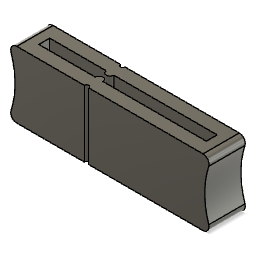
Cassette_Sleeve (Autodesk Fusion 360 design; units mm, degrees)
Autodesk Fusion 360 part; units mm, degrees
sketch "Sketch1" plane through (0, 0, 0) normal (0, 1, 0) x (1, 0, 0)
  line L0 (0, 0) -> (33.75, 0)
  line L1 (33.75, 0) -> (33.75, -6)
  line L2 (33.75, -6) -> (0, -6)
  line L3 (0, -6) -> (0, 0)
  line L4 (3, -3.9) -> (3, -2.1)
  line L5 (30.75, -2.1) -> (30.75, -3.9)
  line L6 (30.75, -3.9) -> (13.625, -3.9)
  line L7 (12.375, -3.9) -> (3, -3.9)
  line L8 (3, -2.1) -> (12.375, -2.1)
  line L9 (13.625, -2.1) -> (30.75, -2.1)
  arc A0 (12.375, -2.1) -> (13.625, -2.1) centre (13, -2.1) ccw
  arc A1 (12.625, 0) -> (13.375, 0) centre (13, 0) ccw
  arc A2 (13.375, -6) -> (12.625, -6) centre (13, -6) ccw
  arc A3 (13.625, -3.9) -> (12.375, -3.9) centre (13, -3.9) ccw
  dimension "d1" = 33.75
  dimension "d2" = 6
  dimension "d8" = 2.1
  dimension "d9" = 3
  dimension "d10" = 2.1
  dimension "d11" = 3
  dimension "d12" = 27
  dimension "d20" = 10
  dimension "d22" = 10
  dimension "d25" = 0.75
  dimension "d26" = 0.75
  dimension "d27" = 0.625
  dimension "d33" = 1.25
  constraint horizontal L0
  constraint vertical L1
  constraint horizontal L2
  constraint vertical L3
  constraint coincident L0.start L3.end
  constraint parallel L2 L6
  constraint parallel L3 L4
  constraint parallel L0 L8
  constraint parallel L1 L5
  constraint coincident L3.end L0
  constraint coincident L0.start L3
  constraint collinear L6 L7
  constraint collinear L8 L9
  constraint coincident L0 A1.centre
  constraint coincident L0 A1.end
  constraint coincident L0 A1.start
  constraint coincident L2 A2.end
  constraint coincident L2 A2.start
  measures "d1" distance of L0.start L0.end
  measures "d2" distance of L0.start L2.end
  measures "d8" distance of L0 L8
  measures "d9" distance of L3 L4
  measures "d10" distance of L2 L6
  measures "d11" distance of L1 L5
  measures "d20" distance of L4 A0.centre
  measures "d22" distance of L4 A3.centre
  measures "d25" diameter of A2
  measures "d26" diameter of A1
  measures "d27" radius of A0
  measures "d33" diameter of A3
extrude "Extrude1" add sketch "Sketch1" along normal blind 11
sketch "Sketch2" plane through (0, 0, 0) normal (0, 0, -1) x (-1, 0, 0)
  line L0 (-33.75, 0) -> (0, 0)
  line L1 (0, 0) -> (0, 11)
  line L2 (0, 11) -> (-33.75, 11)
  line L3 (-33.75, 11) -> (-33.75, 0)
  arc A0 (0, 11) -> (0, 0) centre (12.5393, 5.5) ccw
  line L4 (0, 11) -> (0, 0)
  line L5 (-16.875, 11) -> (-16.875, 0)
  line L6 (-33.75, 11) -> (-33.75, 0)
  arc A1 (-33.75, 0) -> (-33.75, 11) centre (-46.2893, 5.5) ccw
  line L7 (-33.75, 0) -> (-33.75, 11)
  constraint coincident L1.end L2.start
  constraint midpoint L2 L5.start
  constraint midpoint L0 L5.end
  constraint symmetric L0.end L5 L0.start
  constraint symmetric L1.end L5 L2.end
  constraint symmetric A0 L5 A1
extrude "Extrude2" cut sketch "Sketch2" against normal through all contours L3 L6 A1 L7 | L1 A0 L4
fillet "Fillet1" radius 1 2 edges at (0, 11, 3) (0, 0, 3)
fillet "Fillet1" radius 1 2 edges at (33.75, 11, 3) (33.75, 0, 3)
sketch "Sketch3" plane through (0, 11, 0) normal (0, 1, 0) x (-1, 0, 0)
  line L0 (-32.3029, 6) -> (-32.3029, 0)
  line L1 (-32.3029, 0) -> (-1.4471, 0)
  line L2 (-1.4471, 0) -> (-1.4471, 6)
  line L3 (-1.4471, 6) -> (-32.3029, 6)
  line L4 (-30.75, 3.9) -> (-13.625, 3.9)
  line L5 (-3, 3.9) -> (-3, 2.1)
  line L6 (-3, 2.1) -> (-12.375, 2.1)
  arc A0 (-12.375, 2.1) -> (-13.625, 2.1) centre (-13, 2.1) ccw
  line L7 (-13.625, 2.1) -> (-30.75, 2.1)
  line L8 (-30.75, 2.1) -> (-30.75, 3.9)
  circle A1 centre (-13, 0) radius 0.375
  circle A2 centre (-13, 6) radius 0.375
  arc A3 (-13.625, 3.9) -> (-12.375, 3.9) centre (-13, 3.9) ccw
  line L9 (-12.375, 3.9) -> (-3, 3.9)
  dimension "d28" = 0.75
  dimension "d29" = 0.75
  dimension "d30" = 10
  dimension "d31" = 10
  constraint coincident L1 A1.centre
  constraint coincident L3 A2.centre
  measures "d28" diameter of A1
  measures "d29" diameter of A2
  measures "d30" distance of L5 A1.centre
  measures "d31" distance of L5 A2.centre
extrude "Extrude3" cut sketch "Sketch3" against normal through all contours L3 A2 | L1 A1 picked at (-13.0916, 5.915) picked at (-12.9084, 0.085)
equation "d8 = d10"
equation "d11 = d9"
equation "d24 = 0.75 mm"
equation "d25 = d24"
equation "d26 = d24"
equation "d27 = d33 / 2"
equation "d31 = d30"
